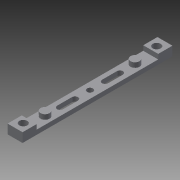
# Autodesk Inventor part: roller_holder
Saved by Autodesk Inventor 2015 (Build 190159000, 159)
## iProperties
Created: 2017-12-04
Part Number: roller_holder
Material: Generic
Document SubType Name: Modeling
Designer: Anshul
Density: 1 g/cm^3
Appearance: Default
Author: Anshul
Autodesk Inventor part; units mm, degrees
ref_plane "YZ Plane" through (0, 0, 0) normal (1, 0, 0) x (0, 1, 0)
ref_plane "XZ Plane" through (0, 0, 0) normal (0, 1, 0) x (-1, 0, 0)
ref_plane "XY Plane" through (0, 0, 0) normal (0, 0, 1) x (1, 0, 0)
sketch "Sketch1" plane through (0, 0, 0) normal (0, 1, 0) x (-1, 0, 0)
  circle A0 centre (0, -20) radius 3
  circle A1 centre (0, -80) radius 3
  circle A2 centre (0, -5.5) radius 2.65
  circle A3 centre (0, -94.5) radius 2.65
  line L0 (0, -100) -> (5, -100)
  line L1 (5, -100) -> (5, 0)
  line L2 (5, 0) -> (0, 0)
  line L3 (0, 0) -> (-5, 0)
  line L4 (-5, 0) -> (-5, -100)
  line L5 (-5, -100) -> (0, -100)
  line L6 (0, -90.5) -> (5, -90.5)
  line L7 (0, -90.5) -> (-5, -90.5)
  line L8 (0, -9.5) -> (5, -9.5)
  line L9 (0, -9.5) -> (-5, -9.5)
  arc A4 (2, -30) -> (-2, -30) centre (0, -30) ccw
  arc A5 (-2, -40) -> (2, -40) centre (0, -40) ccw
  arc A6 (2, -60) -> (-2, -60) centre (0, -60) ccw
  arc A7 (-2, -70) -> (2, -70) centre (0, -70) ccw
  circle A8 centre (0, -50) radius 2
  line L10 (2, -30) -> (2, -40)
  line L11 (-2, -30) -> (-2, -40)
  line L12 (2, -60) -> (2, -70)
  line L13 (-2, -60) -> (-2, -70)
  dimension "d0" = 100
  dimension "d3" = 6
  dimension "d4" = 6
  dimension "d10" = 5.3
  dimension "d11" = 5.3
  dimension "d12" = 5
  dimension "d13" = 5
  dimension "d20" = 4
  dimension "d21" = 4
  dimension "d22" = 4
  dimension "d23" = 4
  dimension "d24" = 4
  constraints: 28 end point, 12 point on line, 9 centre point, 8 point on circle, 5 perpendicular, 2 tangent, 1 horizontal
  measures "d0" distance of L2.end L0.start
  measures "d3" diameter of A0
  measures "d4" diameter of A1
  measures "d10" diameter of A2
  measures "d11" diameter of A3
  measures "d12" distance of L0.start L0.end
  measures "d13" distance of L2.end L3.end
  measures "d20" diameter of A4
  measures "d21" diameter of A5
  measures "d22" diameter of A6
  measures "d23" diameter of A7
  measures "d24" diameter of A8
extrude "Extrusion1" add sketch "Sketch1" along normal blind 3 contours L6 L7 L4 L9 L8 L1
extrude "Extrusion2" add sketch "Sketch1" along normal blind 6.2 contours A0 | A1 | L5 L4 L7 L6 L1 L0 | L8 L9 L4 L3 L2 L1
body "Solid1"
